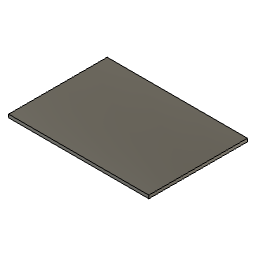
3rd Plate M v2 (Autodesk Fusion 360 design; units mm, degrees)
Autodesk Fusion 360 part; units mm, degrees
sketch "Sketch1" plane through (0, 0, 0) normal (0, 0, 1) x (1, 0, 0)
  line L0 (142.8, -100.4) -> (-142.8, -100.4)
  line L1 (-142.8, -100.4) -> (-142.8, 100.4)
  line L2 (-142.8, 100.4) -> (142.8, 100.4)
  line L3 (142.8, 100.4) -> (142.8, -100.4)
  line L4 (142.8, -100.4) -> (-142.8, 100.4) construction
  line L5 (-142.8, -100.4) -> (142.8, 100.4) construction
  dimension "d1" = 200.8
  dimension "d2" = 285.6
  constraint horizontal L0
  constraint perpendicular L0 L1
  constraint parallel L0 L2
  constraint parallel L1 L3
  constraint coincident L4 origin
  constraint coincident L5 origin
  measures "d1" distance of L0.end L1.end
  measures "d2" distance of L1.end L2.end
extrude "Extrude1" add sketch "Sketch1" along normal blind 6.35
